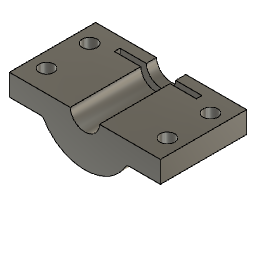
cover_1cc v3 (Autodesk Fusion 360 design; units mm, degrees)
Autodesk Fusion 360 part; units mm, degrees
sketch "スケッチ1" plane through (0, 0, 0) normal (0, 0, 1) x (1, 0, 0)
  line L0 (-19, 20) -> (19, 20)
  line L1 (19, 20) -> (19, 0)
  line L2 (19, 0) -> (-19, 0)
  line L3 (-19, 0) -> (-19, 20)
  dimension "d1" = 38
  dimension "d2" = 20
  constraint horizontal L0
  constraint vertical L1
  constraint horizontal L2
  constraint vertical L3
  constraint midpoint origin L2
  measures "d1" distance of L0.start L0.end
  measures "d2" distance of L0.end L1.end
extrude "押し出し1" add sketch "スケッチ1" along normal blind 15
sketch "スケッチ2" plane through (0, 0, 0) normal (0, -1, 0) x (1, 0, 0)
  line L0 (-19, 0) -> (19, 0)
  line L1 (19, 0) -> (19, 15)
  line L2 (19, 15) -> (-19, 15)
  line L3 (-19, 15) -> (-19, 0)
  line L4 (-19, 15.1531) -> (19, 15.1531) construction
  arc A0 (-3.4, 15.1531) -> (3.4, 15.1531) centre (0, 15.1531) ccw
  line L5 (3.4, 15.1531) -> (3.4, 15)
  line L6 (-3.4, 15.1531) -> (-3.4, 15)
  dimension "d6" = 6.8
  constraint coincident L3 L4.start
  constraint coincident L1 L4.end
  constraint perpendicular L1 L4
  constraint midpoint L4 A0.centre
  constraint coincident L4 A0.end
  constraint coincident L4 A0.start
  constraint coincident L2 L5.end
  constraint tangent A0 L5
  constraint coincident L2 L6.end
  constraint tangent A0 L6
  measures "d6" diameter of A0
extrude "押し出し2" cut sketch "スケッチ2" against normal blind 20 contours L2 A0
ref_plane "WorkPlane2" through (0, 17, 0) normal (0, 1, 0) x (0, 0, 1)
sketch "Sketch5" plane through (0, 17, 0) normal (0, 1, 0) x (1, 0, 0)
  line L0 (0, -9) -> (-9.5, -12.75)
  line L1 (-9.5, -12.75) -> (-9.5, -15)
  line L2 (-9.5, -15) -> (0, -15)
  line L3 (9.5, -15) -> (0, -15)
  line L4 (9.5, -12.75) -> (9.5, -15)
  line L5 (0, -9) -> (9.5, -12.75)
  arc A0 (3.3966, -15) -> (-3.3966, -15) centre (0, -15.1531) ccw
  line L6 (3.3966, -15) -> (19, -15)
  line L7 (19, -15) -> (19, 0)
  line L8 (19, 0) -> (-19, 0)
  line L9 (-19, 0) -> (-19, -15)
  line L10 (-19, -15) -> (-3.3966, -15)
  constraint vertical L1
  constraint perpendicular L1 L2
extrude "Extrude5" cut sketch "Sketch5" along normal blind 0.65 and the other way blind 0.65 contours L0 L1 L2 L3 L4 L5 A0 L6 L10 | L2 L3 A0
sketch "スケッチ4" plane through (0, 0, 15) normal (0, 0, 1) x (-1, 0, 0)
  line L0 (3.3966, -20) -> (19, -20)
  line L1 (19, -20) -> (19, 0)
  line L2 (19, 0) -> (3.3966, 0)
  line L3 (19, -15.125) -> (-17.5478, -15.125) construction
  line L4 (-19, -20) -> (-3.3966, -20) construction
  line L5 (19, -5.125) -> (-19, -5.125) construction
  line L6 (-19, 0) -> (-19, -20) construction
  circle A0 centre (-14, -15.125) radius 1.7
  circle A1 centre (-14, -5.125) radius 1.7
  circle A2 centre (14, -15.125) radius 1.7
  circle A3 centre (14, -5.125) radius 1.7
  line L7 (9.5, -17.65) -> (3.3966, -17.65)
  line L8 (3.3966, -17.65) -> (3.3966, -20)
  line L9 (3.3966, 0) -> (3.3966, -16.35)
  line L10 (3.3966, -16.35) -> (9.5, -16.35)
  line L11 (9.5, -16.35) -> (9.5, -17.65)
  dimension "d15" = 4.875
  dimension "d16" = 10
  dimension "d17" = 3.4
  dimension "d18" = 5
  dimension "d19" = 3.4
  dimension "d20" = 5
  dimension "d21" = 3.4
  dimension "d22" = 5
  dimension "d23" = 3.4
  dimension "d24" = 5
  constraint coincident L1 L3.start
  constraint perpendicular L1 L3
  constraint coincident L1 L5.start
  constraint perpendicular L1 L5
  constraint coincident L5.end L6
  constraint coincident L3 A0.centre
  constraint coincident L5 A1.centre
  constraint coincident L3 A2.centre
  constraint coincident L5 A3.centre
  measures "d15" distance of L3 L4
  measures "d16" distance of L3 L5
  measures "d17" diameter of A0
  measures "d18" distance of L6 A0.centre
  measures "d19" diameter of A1
  measures "d20" distance of L6 A1.centre
  measures "d21" diameter of A2
  measures "d22" distance of L1 A2.centre
  measures "d23" diameter of A3
  measures "d24" distance of L1 A3.centre
extrude "押し出し4" cut sketch "スケッチ4" against normal blind 25 contours A0 | A1 | A2 | A3
sketch "Sketch6" plane through (0, 0, 0) normal (0, -1, 0) x (1, 0, 0)
  arc A0 (-3.3966, 15) -> (3.3966, 15) centre (0, 15.1531) ccw
  line L0 (-3.3966, 15) -> (-19, 15)
  line L1 (-19, 15) -> (-19, 0)
  line L2 (-19, 0) -> (19, 0)
  line L3 (19, 0) -> (19, 15)
  line L4 (19, 15) -> (3.3966, 15)
  circle A1 centre (0, 15.1531) radius 11
  line L5 (-19, 15) -> (19, 15)
  line L6 (19, 15) -> (19, 10)
  line L7 (19, 10) -> (-19, 10)
  line L8 (-19, 10) -> (-19, 15)
  dimension "d32" = 22
  dimension "d33" = 5
  constraint concentric A0 A1
  constraint horizontal L5
  constraint vertical L6
  constraint horizontal L7
  constraint vertical L8
  constraint coincident L3 L6.end
  constraint coincident L0.end L1.start
  measures "d32" diameter of A1
  measures "d33" distance of L0.end L7.end
extrude "Extrude6" cut sketch "Sketch6" against normal blind 25 contours L1 L2 L3 A1 L7
fillet "Fillet1" radius 1 2 edges at (-9.7183, 10, 10) (9.7183, 10, 10)
move_face "OffsetFaces1" offset -1.5 1 faces at (-19, 6.6667, 11.6667)
move_face "OffsetFaces2" offset -1.5 1 faces at (19, 13.3333, 11.6667)
